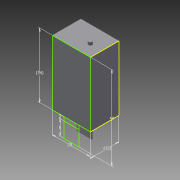
# Autodesk Inventor part: VReg
Saved by Autodesk Inventor 2015 (Build 190159000, 159)
## iProperties
Created: 2014-11-25
Part Number: VReg
Material: Generic
Document SubType Name: Modeling
Designer: s4201025
Density: 1 g/cm^3
Appearance: Default
Author: s4201025
Autodesk Inventor part; units mm, degrees
ref_plane "YZ Plane" through (0, 0, 0) normal (1, 0, 0) x (0, 1, 0)
ref_plane "XZ Plane" through (0, 0, 0) normal (0, 1, 0) x (-1, 0, 0)
ref_plane "XY Plane" through (0, 0, 0) normal (0, 0, 1) x (1, 0, 0)
sketch "Sketch1" plane through (0, 0, 0) normal (0, 1, 0) x (-1, 0, 0)
  line L0 (-10, 34) -> (10, 34)
  line L1 (10, 34) -> (10, 0)
  line L2 (10, 0) -> (-10, 0)
  line L3 (-10, 0) -> (-10, 34)
  line L4 (-4, 0) -> (4, 0)
  line L5 (4, 0) -> (4, -2)
  line L6 (4, -2) -> (-4, -2)
  line L7 (-4, -2) -> (-4, 0)
  line L8 (-4, -2) -> (4, -2)
  line L9 (4, -2) -> (4, -10)
  line L10 (4, -10) -> (-4, -10)
  line L11 (-4, -10) -> (-4, -2)
  dimension "d0" = 20
  dimension "d3" = 2
  dimension "d4" = 8
  dimension "d5" = 44
  dimension "d6" = 34
  constraints: 24 end point, 6 parallel, 3 horizontal, 3 perpendicular, 1 point on line
  measures "d0" distance of L1.end L2.end
  measures "d3" distance of L4.end L5.end
  measures "d4" distance of L8.end L9.end
  measures "d5" distance between parallel lines of L10 L0
  measures "d6" distance between parallel lines of L2 L0
extrude "Extrusion1" add sketch "Sketch1" along normal blind 15 contours L0 L1 L2 L3
extrude "Extrusion2" add sketch "Sketch1" along normal blind 7 contours L2 L5 L6 L7
extrude "Extrusion3" add sketch "Sketch1" along normal blind 7 contours L6 L9 L10 L11
extrude "Extrusion4" cut sketch "Sketch1" along normal blind 8 contours L2 L5 L6 L7
extrude "Extrusion5" add sketch "Sketch1" along normal blind 8 contours L2 L5 L6 L7
extrude "Extrusion6" cut sketch "Sketch1" along normal blind 6 contours L2 L5 L6 L7
extrude "Extrusion7" add sketch "Sketch1" along normal blind 7.25 contours L6 L9 L10 L11
extrude "Extrusion8" cut sketch "Sketch1" along normal blind 6.75 contours L6 L9 L10 L11
sketch "Sketch2" plane through (-10, 0, 34) normal (0, 0, 1) x (1, 0, 0)
  circle A0 centre (14, 6) radius 1
  point P0 (10, 0)
  dimension "d25" = 2
  constraints: 1 centre point
  measures "d25" diameter of A0
extrude "Extrusion9" add sketch "Sketch2" along normal blind 1.5
sketch "Sketch3" plane through (10, 0, 34) normal (1, 0, 0) x (0, 0, -1)
  line L0 (0, 0) -> (34, 0) projected
  line L1 (34, 0) -> (34, 15) projected
  line L2 (0, 15) -> (34, 15) projected
  line L3 (0, 0) -> (0, 15) projected
  dimension "d28" = 15
  measures "d28" distance between parallel lines of L2 L0
sketch "Sketch5" plane through (0, 15, 0) normal (0, 1, 0) x (1, 0, 0)
  point P0 (0, 0)
body "Solid1"
